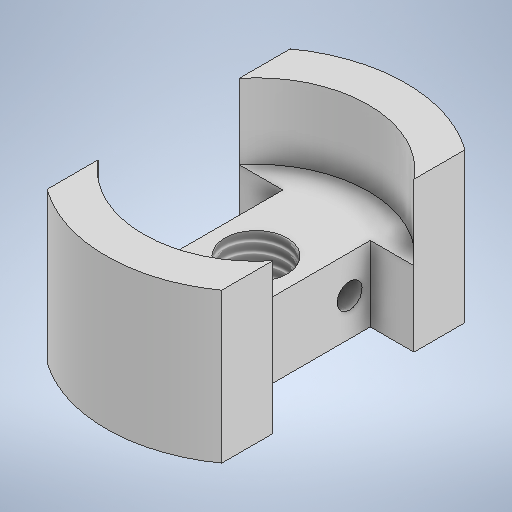
# Autodesk Inventor part: 42
Saved by Autodesk Inventor 2025.1 (Build 291241000, 241)
## iProperties
Created: 2024-09-17
Part Number: 42
Material: Generisch
Document SubType Name: Modeling
Designer: ffogue
Density: 1 g/cm^3
Appearance: Vorgabe
Author: ffogue
Autodesk Inventor part; units mm, degrees
ref_plane "YZ Plane" through (0, 0, 0) normal (1, 0, 0) x (0, 1, 0)
ref_plane "XZ Plane" through (0, 0, 0) normal (0, 1, 0) x (-1, 0, 0)
ref_plane "XY Plane" through (0, 0, 0) normal (0, 0, 1) x (1, 0, 0)
sketch "Sketch1" plane through (0, 0, 0) normal (0, 0, 1) x (1, 0, 0)
  arc A0 (7, 17.6569) -> (-7, 17.6569) centre (0, 12) ccw
  arc A1 (7, 21.7468) -> (-7, 21.7468) centre (0, 12) ccw
  line L0 (-7, 17.6569) -> (-7, 21.7468)
  line L1 (7, 17.6569) -> (7, 21.7468)
  line L2 (-7, 17.6569) -> (-3.5, 17.6569)
  line L3 (-3.5, 17.6569) -> (-3.5, 6.3431)
  line L4 (-3.5, 6.3431) -> (-7, 6.3431)
  line L5 (-7, 6.3431) -> (-7, 2.2532)
  arc A2 (-7, 2.2532) -> (7, 2.2532) centre (0, 12) ccw
  arc A3 (-7, 6.3431) -> (7, 6.3431) centre (0, 12) ccw
  line L6 (7, 6.3431) -> (7, 2.2532)
  line L7 (7, 6.3431) -> (3.5, 6.3431)
  line L8 (3.5, 6.3431) -> (3.5, 17.6569)
  line L9 (3.5, 17.6569) -> (7, 17.6569)
  line L10 (0, 0) -> (0, 24) construction
  line L11 (-10.3169, 12) -> (3.5, 12) construction
  point P0 (0, 3)
  dimension "d4" = 24
  dimension "d5" = 12
  dimension "d6" = 14
  dimension "d7" = 9
  dimension "d8" = 3.5
  dimension "d9" = 12
  dimension "d10" = 7
  dimension "d11" = 3.5
  dimension "d12" = 9
  dimension "d13" = 12
  constraints: 24 end point, 11 point on circle, 5 vertical alignment, 4 centre point, 4 perpendicular, 3 horizontal, 3 symmetric about line, 3 vertical, 2 concentric, 1 midpoint, 1 parallel, 3 other
  measures "d4" distance of L10.start L10.end
  measures "d5" radius of A1
  measures "d6" distance between parallel lines of L6 L5
  measures "d7" radius of A3
  measures "d8" distance from line of L3 L4.end
  measures "d9" distance of L10.start A0.centre
  measures "d10" distance between parallel lines of L10 L5
  measures "d11" distance from line of L6.start L8
  measures "d12" radius of A0
  measures "d13" radius of A2
extrude "Extrusion1" add sketch "Sketch1" along normal blind 6 contours L9 L8 L7 A3 L4 L3 L2 A0
extrude "Extrusion2" add sketch "Sketch1" along normal blind 12 contours A0 L0 A1 L1 | L6 A2 L5 A3
sketch "Sketch2" plane through (0, 0, 6) normal (0, 0, 1) x (1, 0, 0)
  circle A0 centre (0, 12) radius 2.5
  arc A1 (-7, 2.2532) -> (7, 2.2532) centre (0, 12) ccw projected
  point P0 (0, 0)
  point P1 (0, 0)
  point P2 (0, 0)
  dimension "d18" = 12
  dimension "d19" = 5
  constraints: 2 point on circle, 1 centre point, 1 vertical alignment
  measures "d18" distance of point (0, 0) A0.centre
  measures "d19" diameter of A0
extrude "Extrusion3" cut sketch "Sketch2" against normal up to surface (6 mm away)
thread "Thread1" size "M5x0.8" class "6H" standard "ISO Metric profile" full length
sketch "Sketch3" plane through (3.5, 6.3431, 0) normal (1, 0, 0) x (0, 0, -1)
  line L0 (0, 0) -> (0, 11.3137) projected
  point P0 (0, -6.3431)
  point P1 (-3, 1.6569)
  point P2 (-3, 9.6569)
  point P3 (0, 5.6569)
  dimension "d24" = 3
  dimension "d25" = 8
  dimension "d26" = 4
  constraints: 1 midpoint, 1 vertical alignment
  measures "d24" distance from line of L0 point (-3, 1.657)
  measures "d25" distance of point (-3, 9.657) point (-3, 1.657)
  measures "d26" vertical distance of point (0, 5.657) point (-3, 1.657)
hole "Hole1" at (3.5, 8, 3) at (3.5, 16, 3) direction (-1, 0, 0) diameter 2 depth 7
equation "\"d9\" = 0.5 * d4"
equation "\"d26\" = 0.5 * d25"
body "Solid1"
